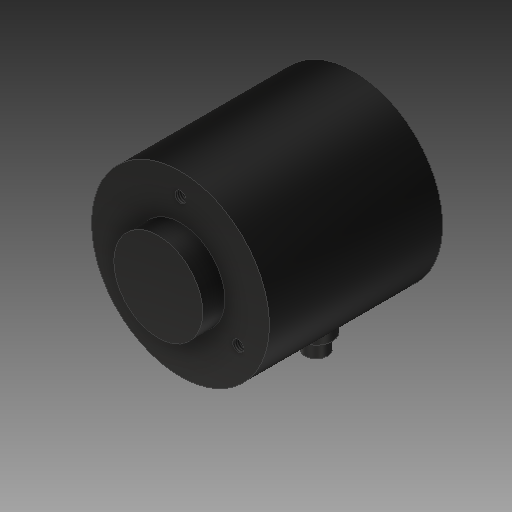
# Autodesk Inventor part: Belt Encoder Body
Saved by Autodesk Inventor 2018 (Build 220112000, 112)
## iProperties
Created: 2017-05-30
Part Number: Belt Encoder Body
Material: ABS Plastic
Document SubType Name: Modeling
Designer: M220404
Density: 1.06 g/cm^3
Appearance: Glossy - Black
Mass: 53.808 g
Surface Area: 84.2844 cm^2
Volume: 50.7622 cm^3
Author: M220404
Autodesk Inventor part; units mm, degrees
ref_plane "YZ Plane" through (0, 0, 0) normal (1, 0, 0) x (0, 1, 0)
ref_plane "XZ Plane" through (0, 0, 0) normal (0, 1, 0) x (-1, 0, 0)
sketch "Sketch1" plane through (0, 0, 0) normal (0, 1, 0) x (-1, 0, 0)
  circle A0 centre (0, 0) radius 20
  dimension "d0" = 40
  constraints: 1 centre point, 1 coincident
  measures "d0" diameter of A0
extrude "Extrusion1" add sketch "Sketch1" along normal blind 39
sketch "Sketch2" plane through (0, 39, 0) normal (0, 1, 0) x (1, 0, 0)
  circle A0 centre (0, 0) radius 10
  dimension "d3" = 20
  constraints: 1 centre point, 1 coincident
  measures "d3" diameter of A0
extrude "Extrusion2" add sketch "Sketch2" along normal blind 5
sketch "Sketch3" plane through (0, 39, 0) normal (0, 1, 0) x (1, 0, 0)
  circle A0 centre (0, 0) radius 15 construction
  circle A1 centre (0, 0) radius 20 construction
  point P0 (0, 15)
  point P1 (-12.9904, -7.5)
  point P2 (12.9904, -7.5)
  dimension "d6" = 30
  dimension "d9" = 360
  constraints: 1 coincident, 1 vertical alignment, 6 other
hole "Hole1" at (0, 39, -15) at (-12.9904, 39, 7.5) at (12.9904, 39, 7.5) direction (0, -1, 0) diameter 2.459 depth 9.8 tip angle 118 thread size "M3x0.5" class "6H" standard "ANSI Metric M Profile"
ref_plane "Work Plane2" through (0, 0, 20) normal (0, 0, 1) x (1, 0, 0)
sketch "Sketch6" plane through (0, 0, 20) normal (0, 0, 1) x (1, 0, 0)
  line L0 (20, 39) -> (-20, 39) projected
  line L1 (-20, 0) -> (20, 0) projected
  line L2 (-20, 0) -> (-20, 39) projected
  line L3 (20, 0) -> (20, 39) projected
  circle A0 centre (0, 8.47) radius 3.65
  circle A1 centre (0, 8.47) radius 2.75
  point P0 (0, 0)
  dimension "d25" = 7.3
  dimension "d26" = 8.47
  dimension "d29" = 0.9
  constraints: 2 centre point
  measures "d25" diameter of A0
  measures "d26" distance from line of L1 A0.centre
  measures "d29" radial gap between concentric circles of A0 A1
extrude "Extrusion6" add sketch "Sketch6" along normal blind 6.58 and the other way blind 3.29 contours A0
sketch "Sketch7" plane through (0, 0, 20) normal (0, 0, 1) x (1, 0, 0)
  line L0 (20, 39) -> (-20, 39) projected
  line L1 (-20, 0) -> (-20, 39) projected
  line L2 (-20, 0) -> (20, 0) projected
  line L3 (20, 0) -> (20, 39) projected
  arc A0 (0, 4.82) -> (0, 12.12) centre (0, 8.47) ccw projected
  circle A1 centre (0, 8.47) radius 2.55
  point P0 (0, 0)
  dimension "d32" = 5.1
  constraints: 2 coincident, 1 centre point
  measures "d32" diameter of A1
extrude "Extrusion7" add sketch "Sketch7" along normal blind 10 contours A1
body "Solid1"
